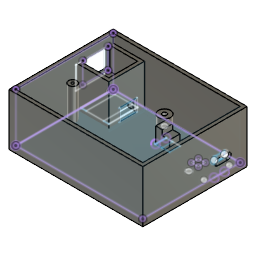
blindaphone box v2 bottom (Autodesk Fusion 360 design; units mm, degrees)
part number: 2026-05-01-20-35-57-796
Autodesk Fusion 360 part; units mm, degrees
note: some values were not read from the file. Set by a fixed rule: which face or edge a step refers to.
sketch "Sketch2" plane through (0, 0, 0) normal (0, 0, 1) x (1, 0, 0)
  line L0 (38.5, -30) -> (-38.5, -30)
  line L1 (-38.5, -30) -> (-38.5, 30)
  line L2 (-38.5, 30) -> (38.5, 30)
  line L3 (38.5, 30) -> (38.5, -30)
  line L4 (38.5, -30) -> (-38.5, 30) construction
  line L5 (-38.5, -30) -> (38.5, 30) construction
  dimension "d3" = 77
  dimension "d4" = 60
  constraint horizontal L0
  constraint perpendicular L0 L1
  constraint parallel L0 L2
  constraint parallel L1 L3
  constraint coincident L4 origin
  constraint coincident L5 origin
  measures "d3" distance of L1.end L2.end
  measures "d4" distance of L0.end L1.end
extrude "Extrude1" add sketch "Sketch2" along normal blind 30 makes body 1
shell "Shell1" thickness 2 removed faces 1 at (-12.8333, 10, 30) on bodies 1
sketch "Sketch14" plane through (0, 0, 2) normal (0, 0, 1) x (-1, 0, 0)
  line L0 (-36.5, -28) -> (36.5, -28)
  line L1 (36.5, -28) -> (36.5, 28)
  line L2 (36.5, 28) -> (-36.5, 28)
  line L3 (-36.5, 28) -> (-36.5, -28)
  line L4 (36.5, -26) -> (20.5, -26)
  line L5 (20.5, -26) -> (20.5, -9.5)
  line L6 (20.5, -9.5) -> (36.5, -9.5)
  line L7 (36.5, -9.5) -> (36.5, -26)
  line L8 (36.5, -26) -> (33.5, -26)
  line L9 (33.5, -26) -> (33.5, -9.5)
  line L10 (33.5, -9.5) -> (36.5, -9.5)
  line L11 (36.5, -9.5) -> (36.5, -26)
  line L12 (20.5, -26) -> (23.5, -26)
  line L13 (23.5, -26) -> (23.5, -9.5)
  line L14 (23.5, -9.5) -> (20.5, -9.5)
  line L15 (20.5, -9.5) -> (20.5, -26)
  dimension "d125" = 16
  dimension "d126" = 16.5
  dimension "d130" = 2
  dimension "d131" = 3
  dimension "d132" = 3
  constraint horizontal L4
  constraint vertical L5
  constraint horizontal L6
  constraint vertical L7
  constraint coincident L1 L4.start
  constraint horizontal L8
  constraint vertical L9
  constraint horizontal L10
  constraint vertical L11
  constraint horizontal L12
  constraint vertical L13
  constraint horizontal L14
  constraint vertical L15
  measures "d125" distance of L4.start L4.end
  measures "d126" distance of L4.start L6.end
  measures "d130" distance of L0 L4
  measures "d131" distance of L4.start L8.end
  measures "d132" distance of L4.end L12.end
extrude "Extrude18" add sketch "Sketch14" along normal blind 23 separate body contours L1 L4 L6 L7 L8 L9 L10 L11 | L4 L6 L9 L13 | L4 L5 L6 L12 L13 L14 L15 makes body 2
shell "Shell8" thickness 2 outward yes removed faces 1 at (-30.1667, 20.5, 25) on bodies 2
extrude "Extrude19" add sketch "Sketch14" along normal blind 10 separate body contours L1 L4 L6 L7 L8 L9 L10 L11 | L4 L5 L6 L12 L13 L14 L15 makes body 3 at (-33.5, 20.5, 8.6667) makes body 4 at (-20.5, 20.5, 8.6667)
sketch "Sketch15" plane through (-18.5, 0, 0) normal (1, 0, 0) x (0, 1, 0)
  line L0 (7.5, 0) -> (28, 0)
  line L1 (28, 0) -> (28, 25)
  line L2 (28, 25) -> (7.5, 25)
  line L3 (7.5, 25) -> (7.5, 0)
  line L4 (23.5, 2) -> (13.5, 2)
  line L5 (13.5, 2) -> (13.5, 9)
  line L6 (13.5, 9) -> (23.5, 9)
  line L7 (23.5, 9) -> (23.5, 2)
  dimension "d135" = 10
  dimension "d136" = 7
  dimension "d137" = 4.5
  constraint horizontal L4
  constraint vertical L5
  constraint horizontal L6
  constraint vertical L7
  measures "d135" distance of L4.start L4.end
  measures "d136" distance of L4.start L6.end
  measures "d137" distance of L1 L7
extrude "Extrude20" cut sketch "Sketch15" against normal blind 7.5 contours L4 L5 L6 L7 bodies 2 4
sketch "Sketch16" plane through (-36.5, 0, 0) normal (1, 0, 0) x (0, 1, 0)
  line L0 (9.5, 2) -> (26, 2)
  line L1 (26, 2) -> (26, 25)
  line L2 (26, 25) -> (9.5, 25)
  line L3 (9.5, 25) -> (9.5, 2)
  line L4 (25, 24.99) -> (10.5, 24.99)
  line L5 (10.5, 24.99) -> (10.5, 12.99)
  line L6 (10.5, 12.99) -> (25, 12.99)
  line L7 (25, 12.99) -> (25, 24.99)
  dimension "d140" = 14.5
  dimension "d141" = 12
  dimension "d142" = 1
  dimension "d143" = 0.01
  constraint horizontal L4
  constraint vertical L5
  constraint horizontal L6
  constraint vertical L7
  measures "d140" distance of L4.start L4.end
  measures "d141" distance of L4.start L6.end
  measures "d142" distance of L1 L7
  measures "d143" distance of L2 L4
extrude "Extrude21" cut sketch "Sketch16" against normal blind 4 contours L4 L5 L6 L7 bodies 1 2
sketch "Sketch3" plane through (-36.5, 0, 0) normal (1, 0, 0) x (0, 1, 0)
  line L0 (-28, 2) -> (28, 2)
  line L1 (28, 2) -> (28, 30)
  line L2 (28, 30) -> (-28, 30)
  line L3 (-28, 30) -> (-28, 2)
  line L4 (6.5, 25) -> (23, 25)
  line L5 (23, 25) -> (23, 12)
  line L6 (23, 12) -> (6.5, 12)
  line L7 (6.5, 12) -> (6.5, 25)
  line L8 (10.5, 24.99) -> (25, 24.99)
  line L9 (25, 24.99) -> (25, 12.99)
  line L10 (25, 12.99) -> (10.5, 12.99)
  line L11 (10.5, 12.99) -> (10.5, 24.99)
  dimension "d19" = 16.5
  dimension "d20" = 13
  dimension "d123" = 5
  dimension "d124" = 10
  constraint horizontal L4
  constraint vertical L5
  constraint horizontal L6
  constraint vertical L7
  measures "d19" distance of L4.start L4.end
  measures "d20" distance of L4.start L6.end
  measures "d123" distance of L1 L5
  measures "d124" distance of L0 L6
ref_plane "WorkPlane1" through (0, 0, 15) normal (1, 0, 0) x (0, 1, 0)
sketch "Sketch4" plane through (0, 0, 2) normal (0, 0, 1) x (-1, 0, 0)
  line L0 (-36.5, -28) -> (36.5, -28)
  line L1 (36.5, -28) -> (36.5, 28)
  line L2 (36.5, 28) -> (-36.5, 28)
  line L3 (-36.5, 28) -> (-36.5, -28)
  circle A0 centre (33.3, 25) radius 0.9
  circle A1 centre (33.3, -1.5) radius 0.9
  circle A2 centre (-33.3, 25) radius 0.9
  circle A3 centre (-33.3, -1.5) radius 0.9
  dimension "d34" = 1.8
  dimension "d35" = 1.8
  dimension "d36" = 1.8
  dimension "d37" = 1.8
  dimension "d38" = 26.5
  dimension "d39" = 26.5
  dimension "d40" = 66.6
  dimension "d41" = 66.6
  dimension "d42" = 3
  dimension "d43" = 3
  dimension "d106" = 3.2
  dimension "d107" = 3.2
  measures "d34" diameter of A0
  measures "d35" diameter of A1
  measures "d36" diameter of A2
  measures "d37" diameter of A3
  measures "d38" vertical distance of A0.centre A1.centre
  measures "d39" vertical distance of A2.centre A3.centre
  measures "d40" distance of A0.centre A2.centre
  measures "d41" distance of A1.centre A3.centre
  measures "d42" distance of L2 A0.centre
  measures "d43" distance of L2 A2.centre
  measures "d106" distance of L3 A3.centre
  measures "d107" distance of L3 A2.centre
extrude "Extrude6" add sketch "Sketch4" along normal blind 18 separate body contours A0 | A1 | A2 | A3 makes body 5 at (-33.6702, 2.3204, 14) makes body 6 at (32.8894, -25.8009, 14) makes body 7 at (-33.7106, -25.8009, 14) makes body 8 at (32.9298, 2.3204, 14)
shell "Shell4" thickness 1.5 outward yes removed faces 4 at (-33.3219, 1.2075, 20) at (33.3239, -25.2793, 20) at (-33.3668, -24.7075, 20) at (32.6598, 1.6859, 20) on bodies 5 6 7 8
thread "Thread1" "ISO Metric profile 1.8 M1.8x0.35 M1.8x0.35 6H" major diameter 1.8678 minor diameter 1.4711 pitch 0.35 angle 60 resizes the face on face at (32.9298, 2.3204, 14) from (33.3, 1.5, 14) to (33.3, 1.5, 20) on face at (-33.7106, -25.8009, 14) from (-33.3, -25, 14) to (-33.3, -25, 20) on face at (-33.6702, 2.3204, 14) from (-33.3, 1.5, 14) to (-33.3, 1.5, 20) on face at (32.8894, -25.8009, 14) from (33.3, -25, 14) to (33.3, -25, 20) on bodies 5 6 7 8
sketch "Sketch6" plane through (0, 0, 2) normal (0, 0, 1) x (-1, 0, 0)
  line L0 (-36.5, -28) -> (36.5, -28)
  line L1 (36.5, -28) -> (36.5, 28)
  line L2 (36.5, 28) -> (-36.5, 28)
  line L3 (-36.5, 28) -> (-36.5, -28)
  circle A0 centre (-34.7, -23.5) radius 0.9
  circle A1 centre (-34.7, -9) radius 0.9
  line L4 (-2.9, -19) -> (-2.9, -13)
  line L5 (-10.9, -19) -> (-2.9, -19)
  line L6 (-2.9, -19) -> (-2.9, -13)
  line L7 (-2.9, -13) -> (-10.9, -13)
  line L8 (-10.9, -13) -> (-10.9, -19)
  line L9 (-2.9, -19) -> (-6.7, -19)
  line L10 (-6.7, -19) -> (-6.7, -13)
  line L11 (-6.7, -13) -> (-2.9, -13)
  line L12 (-2.9, -13) -> (-2.9, -19)
  line L13 (-22.5, -18) -> (-26.5, -18)
  line L14 (-26.5, -18) -> (-26.5, -14)
  line L15 (-26.5, -14) -> (-22.5, -14)
  line L16 (-22.5, -14) -> (-22.5, -18)
  dimension "d52" = 1.8
  dimension "d53" = 1.8
  dimension "d54" = 4.5
  dimension "d55" = 14.5
  dimension "d56" = 1.8
  dimension "d57" = 1.8
  dimension "d64" = 8
  dimension "d70" = 3.8
  dimension "d108" = 4
  dimension "d109" = 4
  dimension "d110" = 10
  dimension "d111" = 9
  dimension "d112" = 10
  constraint vertical L4
  constraint horizontal L5
  constraint vertical L6
  constraint horizontal L7
  constraint vertical L8
  constraint horizontal L9
  constraint vertical L10
  constraint horizontal L11
  constraint vertical L12
  constraint horizontal L13
  constraint vertical L14
  constraint horizontal L15
  constraint vertical L16
  measures "d52" diameter of A0
  measures "d53" diameter of A1
  measures "d54" distance of L0 A0.centre
  measures "d55" vertical distance of A0.centre A1.centre
  measures "d56" distance of L3 A0.centre
  measures "d57" distance of L3 A1.centre
  measures "d64" distance of L4 L8
  measures "d70" distance of L4.start L9.end
  measures "d108" distance of L13.start L13.end
  measures "d109" distance of L13.start L15.end
  measures "d110" distance of L3 L14
  measures "d111" distance of L0 L5
  measures "d112" distance of L0 L13
extrude "Extrude7" add sketch "Sketch6" along normal blind 6 separate body contours A0 | A1 | L4 L5 L6 L7 L9 L10 L11 L12 | L5 L7 L8 L10 makes body 9 at (8.2333, 19, 4) makes body 10 at (34.3298, 22.6796, 6) makes body 11 at (34.6776, 8.1003, 6)
shell "Shell5" thickness 1 outward yes removed faces 2 at (34.7668, 23.2075, 8) at (34.6781, 8.7075, 8) on bodies 10 11
thread "Thread3" "ISO Metric profile 1.8 M1.8x0.35 M1.8x0.35 6H" major diameter 1.8678 minor diameter 1.4711 pitch 0.35 angle 60 resizes the face on face at (34.3298, 22.6796, 6) from (34.7, 23.5, 3) to (34.7, 23.5, 8) on face at (34.6776, 8.1003, 6) from (34.7, 9, 3) to (34.7, 9, 8) on bodies 10 11
extrude "Extrude8" add sketch "Sketch6" along normal blind 9 contours L4 L5 L6 L7 L9 L10 L11 L12 bodies 9
extrude "Extrude16" add sketch "Sketch6" along normal blind 6 contours L13 L14 L15 L16 bodies 1
sketch "Sketch7" plane through (0, 0, 2) normal (0, 0, 1) x (-1, 0, 0)
  line L0 (-36.5, -28) -> (36.5, -28)
  line L1 (36.5, -28) -> (36.5, 28)
  line L2 (36.5, 28) -> (-36.5, 28)
  line L3 (-36.5, 28) -> (-36.5, -28)
  circle A0 centre (-26, -9) radius 1.5
  line L4 (-2.9, -19) -> (-2.9, -13)
  line L5 (-36.5, -28) -> (36.5, -28)
  circle A1 centre (3.5, -24.5) radius 1.5
  line L6 (-22.5, -14) -> (-22.5, -18)
  line L7 (-22.5, -18) -> (-26.5, -18)
  line L8 (-26.5, -18) -> (-26.5, -14)
  line L9 (-26.5, -14) -> (-22.5, -14)
  line L10 (36.5, -28) -> (36.5, 28)
  dimension "d73" = 3
  dimension "d76" = 3
  dimension "d77" = 3.5
  dimension "d78" = 29.5
  dimension "d115" = 15.5
  dimension "d117" = 33
  measures "d73" diameter of A0
  measures "d76" diameter of A1
  measures "d77" distance of L0 A1.centre
  measures "d78" horizontal distance of A0.centre A1.centre
  measures "d115" vertical distance of A0.centre A1.centre
  measures "d117" distance of A1.centre L10
extrude "Extrude17" add sketch "Sketch7" along normal blind 6 separate body contours A0 | A1 makes body 12 at (24.5019, 9.0748, 6) makes body 13 at (-4.9981, 24.5748, 6)
shell "Shell7" thickness 2 outward yes removed faces 2 at (25.5429, 9.5731, 8) at (-3.0166, 24.5729, 8) on bodies 12 13
thread "Thread5" "ISO Metric profile 3.0 M3x0.5 M3x0.5 6H" major diameter 3.086 minor diameter 2.529 pitch 0.5 angle 60 resizes the face on face at (24.5019, 9.0748, 6) from (26, 9, 3) to (26, 9, 8) on face at (-4.9981, 24.5748, 6) from (-3.5, 24.5, 3) to (-3.5, 24.5, 8) on bodies 12 13
sketch "Sketch9" plane through (36.5, 0, 0) normal (-1, 0, 0) x (0, -1, 0)
  line L0 (-28, 2) -> (28, 2)
  line L1 (28, 2) -> (28, 30)
  line L2 (28, 30) -> (-28, 30)
  line L3 (-28, 30) -> (-28, 2)
  circle A0 centre (-19, 10.7) radius 1.5
  circle A1 centre (-13, 10.7) radius 1.5
  line L4 (-13, 2) -> (-19, 2)
  line L5 (-19, 12.2) -> (-13, 12.2)
  line L6 (-13, 12.2) -> (-13, 9.2)
  line L7 (-13, 9.2) -> (-19, 9.2)
  line L8 (-19, 9.2) -> (-19, 12.2)
  circle A2 centre (-19, 10.7) radius 1.8
  circle A3 centre (-13, 10.7) radius 1.8
  line L9 (-19, 12.5) -> (-12.9659, 12.5)
  line L10 (-12.9659, 12.5) -> (-12.9659, 8.9003)
  line L11 (-12.9659, 8.9003) -> (-19, 8.9003)
  line L12 (-19, 8.9003) -> (-19, 12.5)
  dimension "d84" = 3
  dimension "d85" = 9
  dimension "d86" = 3
  dimension "d87" = 6
  dimension "d88" = 8.7
  dimension "d89" = 3.6
  dimension "d90" = 3.6
  constraint horizontal L5
  constraint vertical L6
  constraint horizontal L7
  constraint vertical L8
  constraint coincident A1 L6.end
  constraint coincident A0 L5.start
  constraint concentric A0 A2
  constraint concentric A1 A3
  constraint horizontal L9
  constraint vertical L10
  constraint horizontal L11
  constraint vertical L12
  constraint coincident A3 L10.end
  constraint coincident A2 L9.start
  measures "d84" diameter of A0
  measures "d85" distance of L3 A0.centre
  measures "d86" diameter of A1
  measures "d87" distance of A0.centre A1.centre
  measures "d88" distance of A0.centre L4
  measures "d89" diameter of A2
  measures "d90" diameter of A3
extrude "Extrude10" cut sketch "Sketch9" against normal blind 3 contours A0 L8 L12 | A0 L5 L7 A2 | A0 L8 L12 | L5 A2 L12 | A0 A2 L12 | L7 A2 L12 | L7 A2 A3 L11 | A1 A3 L10 | L5 A2 A3 L9 | L5 L7 A2 A3 | A1 L5 A3 L10 | A1 L5 L7 A3 | A1 L7 A3 L10 | A1 L6 | A1 L6 L10 | A1 L10 bodies 1
extrude "Extrude9" add sketch "Sketch7" along normal blind 6 separate body contours A0 | A1 makes body 14 at (24.5019, 9.0748, 6) makes body 15 at (-4.9981, 24.5748, 6)
shell "Shell6" thickness 2 outward yes removed faces 2 at (25.5429, 9.5731, 8) at (-3.0166, 24.5729, 8) on bodies 14 15
thread "Thread4" "ISO Metric profile 3.0 M3x0.5 M3x0.5 6H" major diameter 3.086 minor diameter 2.529 pitch 0.5 angle 60 resizes the face on face at (-4.9981, 24.5748, 6) from (-3.5, 24.5, 2) to (-3.5, 24.5, 8) on face at (24.5019, 9.0748, 6) from (26, 9, 2) to (26, 9, 8) on bodies 14 15
hidden bodies 10 11 14 15
